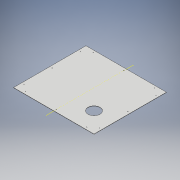
# Autodesk Inventor part: PLEXI 1
Saved by Autodesk Inventor 2018 (Build 220112000, 112)
## iProperties
Created: 2020-08-14
Part Number: PLEXI 1
Material: Ogólny
Document SubType Name: Modeling
Designer: wojwo
Density: 1 g/cm^3
Appearance: Domyślna
Author: wojwo
Autodesk Inventor part; units mm, degrees
ref_plane "YZ Plane" through (0, 0, 0) normal (1, 0, 0) x (0, 1, 0)
ref_plane "XZ Plane" through (0, 0, 0) normal (0, 1, 0) x (-1, 0, 0)
ref_plane "XY Plane" through (0, 0, 0) normal (0, 0, 1) x (1, 0, 0)
sketch "Szkic1" plane through (0, 0, 0) normal (0, 0, 1) x (1, 0, 0)
  line L0 (500, -450) -> (-500, -450)
  line L1 (-500, -450) -> (-500, 450)
  line L2 (-500, 450) -> (500, 450)
  line L3 (500, 450) -> (500, -450)
  line L4 (500, -450) -> (-500, 450) construction
  line L5 (-500, -450) -> (500, 450) construction
  circle A0 centre (250, -200) radius 75
  line L6 (505, -455) -> (-505, -455) construction
  line L7 (-505, -455) -> (-505, 455) construction
  line L8 (-505, 455) -> (505, 455) construction
  line L9 (505, 455) -> (505, -455) construction
  line L10 (505, -455) -> (-505, 455) construction
  line L11 (-505, -455) -> (505, 455) construction
  line L12 (480, -430) -> (-480, -430) construction
  line L13 (-480, -430) -> (-480, 430) construction
  line L14 (-480, 430) -> (480, 430) construction
  line L15 (480, 430) -> (480, -430) construction
  line L16 (480, -430) -> (-480, 430) construction
  line L17 (-480, -430) -> (480, 430) construction
  circle A1 centre (-470, 0) radius 3
  circle A2 centre (-470, 350) radius 3
  circle A3 centre (-470, -350) radius 3
  circle A4 centre (-470, 0) radius 3
  line L18 (0, -722.0928) -> (0, 703.6821) projected
  line L19 (480, -430) -> (480, 430) construction
  circle A5 centre (470, 350) radius 3
  circle A6 centre (470, -350) radius 3
  circle A7 centre (470, 0) radius 3
  circle A8 centre (0, 420) radius 3
  circle A9 centre (380, 420) radius 3
  circle A10 centre (-380, 420) radius 3
  circle A11 centre (0, 420) radius 3
  line L20 (-763, 0) -> (763, 0) projected
  circle A12 centre (0, -420) radius 3
  circle A13 centre (380, -420) radius 3
  circle A14 centre (-380, -420) radius 3
  line L21 (545, -500) -> (-545, -500) construction
  line L22 (-545, -500) -> (-545, 500) construction
  line L23 (-545, 500) -> (545, 500) construction
  line L24 (545, 500) -> (545, -500) construction
  line L25 (545, -500) -> (-545, 500) construction
  line L26 (-545, -500) -> (545, 500) construction
  line L27 (-372.8845, -485.3907) -> (-256.6542, -485.3907) construction
  line L28 (-256.6542, -485.3907) -> (-256.6542, -518.4107) construction
  line L29 (-256.6542, -518.4107) -> (-372.8845, -518.4107) construction
  line L30 (-372.8845, -518.4107) -> (-372.8845, -485.3907) construction
  point P0 (0, 0)
  dimension "d0" = 1000
  dimension "d1" = 900
  dimension "d2" = 150
  dimension "d3" = 250
  dimension "d4" = 250
  dimension "d5" = 1010
  dimension "d6" = 910
  dimension "d7" = 25
  dimension "d8" = 25
  dimension "d9" = 6
  dimension "d10" = 10
  dimension "d13" = 350
  dimension "d16" = 350
  dimension "d19" = 6
  dimension "d20" = 10
  dimension "d23" = 380
  dimension "d26" = 380
  dimension "d31" = 1090
  dimension "d32" = 1000
  constraints: 50 end point, 15 centre point, 8 midpoint, 8 parallel, 6 horizontal, 6 symmetric about line, 4 perpendicular, 2 vertical, 1 point on line, 20 other
  measures "d0" distance of L1.end L2.end
  measures "d1" distance of L0.end L1.end
  measures "d2" diameter of A0
  measures "d3" distance from line of L0 A0.centre
  measures "d4" distance from line of L3 A0.centre
  measures "d5" distance of L7.end L8.end
  measures "d6" distance of L6.end L7.end
  measures "d7" distance between parallel lines of L8 L14
  measures "d8" distance between parallel lines of L7 L13
  measures "d9" diameter of A1
  measures "d10" distance from line of L13 A1.centre
  measures "d13" distance of A1.centre A2.centre
  measures "d16" distance of A1.centre A3.centre
  measures "d19" diameter of A8
  measures "d20" distance from line of L14 A8.centre
  measures "d23" distance of A8.centre A9.centre
  measures "d26" distance of A8.centre A10.centre
  measures "d31" distance of L22.end L23.end
  measures "d32" distance of L21.end L22.end
extrude "Wyciągnięcie proste1" add sketch "Szkic1" along normal blind 3 contours L0 L18 A12 L20 A7 L3 | L0 L1 L20 A1 L18 A12 | L20 A7 L18 A8 L2 L3 | L1 L2 L18 A8 L20 A1
